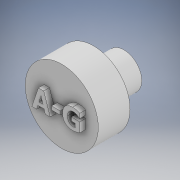
# Autodesk Inventor part: IPC A-G key
Saved by Autodesk Inventor 2022 (Build 260153000, 153)
## iProperties
Created: 2022-01-01
Part Number: IPC A-G key
Material: Generic
Document SubType Name: Modeling
Designer: solor
Density: 1 g/cm^3
Appearance: Default
Author: solor
Autodesk Inventor part; units mm, degrees
ref_plane "YZ Plane" through (0, 0, 0) normal (1, 0, 0) x (0, 1, 0)
ref_plane "XZ Plane" through (0, 0, 0) normal (0, 1, 0) x (-1, 0, 0)
ref_plane "XY Plane" through (0, 0, 0) normal (0, 0, 1) x (1, 0, 0)
sketch "Sketch1" plane through (0, 0, 0) normal (0, 0, 1) x (1, 0, 0)
  circle A0 centre (0, 0) radius 6.22 construction
  circle A1 centre (0, 0) radius 2.8
  line L0 (-0.675, 0.675) -> (-0.675, 2.025)
  line L1 (-0.675, 2.025) -> (0.675, 2.025)
  line L2 (0.675, 2.025) -> (0.675, 0.675)
  line L3 (0.675, 0.675) -> (2.025, 0.675)
  line L4 (2.025, 0.675) -> (2.025, -0.675)
  line L5 (2.025, -0.675) -> (0.675, -0.675)
  line L6 (0.675, -0.675) -> (0.675, -2.025)
  line L7 (0.675, -2.025) -> (-0.675, -2.025)
  line L8 (-0.675, -2.025) -> (-0.675, -0.675)
  line L9 (-0.675, -0.675) -> (-2.025, -0.675)
  line L10 (-2.025, -0.675) -> (-2.025, 0.675)
  line L11 (-2.025, 0.675) -> (-0.675, 0.675)
  circle A2 centre (0, 0) radius 5.75
  point P0 (-6.07, -6.1)
  dimension "d0" = 12.44
  dimension "d1" = 0.47
  constraints: 24 end point, 3 centre point, 1 coincident
  measures "d0" diameter of A0
  measures "d1" radial gap between concentric circles of A0 A2
extrude "Extrusion1" add sketch "Sketch1" along normal blind 5 contours A1 | L0 L1 L2 L3 L4 L5 L6 L7 L8 L9 L10 L11 | A2
extrude "Extrusion2" add sketch "Sketch1" against normal blind 4.8 contours A1
sketch "Sketch2" plane through (0, 0, 5) normal (0, 0, 1) x (1, 0, 0)
  point P0 (0, 0)
sketch "Sketch3" plane through (0, 0, 5) normal (0, 0, 1) x (1, 0, 0)
  line L0 (-3.7906, 1.642) -> (3.8677, 1.642) construction
  line L1 (3.8677, 1.642) -> (3.8677, -1.5876) construction
  line L2 (3.8677, -1.5876) -> (-3.7906, -1.5876) construction
  line L3 (-3.7906, -1.5876) -> (-3.7906, 1.642) construction
  line L4 (-3.803, -1.4674) -> (-2.7723, 1.5826)
  line L5 (-2.7723, 1.5826) -> (-1.9369, 1.5826)
  line L6 (-1.9369, 1.5826) -> (-0.9062, -1.4674)
  line L7 (-0.9062, -1.4674) -> (-1.6947, -1.4674)
  line L8 (-1.6947, -1.4674) -> (-1.885, -0.8445)
  line L9 (-1.885, -0.8445) -> (-2.844, -0.8445)
  line L10 (-2.844, -0.8445) -> (-3.0368, -1.4674)
  line L11 (-3.0368, -1.4674) -> (-3.803, -1.4674)
  line L12 (-2.0531, -0.2909) -> (-2.3645, 0.7176)
  line L13 (-2.3645, 0.7176) -> (-2.6784, -0.2909)
  line L14 (-2.6784, -0.2909) -> (-2.0531, -0.2909)
  line L15 (0.6633, -0.4046) -> (-0.6937, -0.4046)
  line L16 (-0.6937, -0.4046) -> (-0.6937, 0.1639)
  line L17 (-0.6937, 0.1639) -> (0.6633, 0.1639)
  line L18 (0.6633, 0.1639) -> (0.6633, -0.4046)
  spline S0 degree 2 poles (3.7528, -1.2944) (3.5526, -1.3759) (2.9125, -1.5316) (2.601, -1.5316) knots 0 0 0 1 2 2 2
  spline S1 degree 2 poles (2.601, -1.5316) (1.8818, -1.5316) (1.0291, -0.7012) (1.0291, 0.0601) knots 0 0 0 1 2 2 2
  spline S2 degree 2 poles (1.0291, 0.0601) (1.0291, 0.7769) (1.8818, 1.642) (2.6233, 1.642) knots 0 0 0 1 2 2 2
  spline S3 degree 2 poles (2.6233, 1.642) (3.0064, 1.642) (3.4859, 1.4961) (3.7405, 1.3725) knots 0 0 0 1 2 2 2
  line L19 (3.7405, 1.3725) -> (3.7405, 0.6558)
  line L20 (3.7405, 0.6558) -> (3.6712, 0.6558)
  spline S4 degree 2 poles (3.6712, 0.6558) (3.6169, 0.6978) (3.4093, 0.8584) (3.3104, 0.9128) knots 0 0 0 1 2 2 2
  spline S5 degree 2 poles (3.3104, 0.9128) (3.1967, 0.9796) (2.8952, 1.0735) (2.7271, 1.0735) knots 0 0 0 1 2 2 2
  spline S6 degree 2 poles (2.7271, 1.0735) (2.5318, 1.0735) (2.208, 0.9499) (2.082, 0.8238) knots 0 0 0 1 2 2 2
  spline S7 degree 2 poles (2.082, 0.8238) (1.9609, 0.7003) (1.82, 0.3221) (1.82, 0.0725) knots 0 0 0 1 2 2 2
  spline S8 degree 2 poles (1.82, 0.0725) (1.82, -0.4614) (2.3563, -0.9706) (2.8185, -0.9706) knots 0 0 0 1 2 2 2
  spline S9 degree 2 poles (2.8185, -0.9706) (2.8606, -0.9706) (2.9693, -0.9656) (3.0113, -0.9632) knots 0 0 0 1 2 2 2
  line L21 (3.0113, -0.9632) -> (3.0113, -0.3625)
  line L22 (3.0113, -0.3625) -> (2.4206, -0.3625)
  line L23 (2.4206, -0.3625) -> (2.4206, 0.2084)
  line L24 (2.4206, 0.2084) -> (3.7528, 0.2084)
  line L25 (3.7528, 0.2084) -> (3.7528, -1.2944)
  point P0 (0.0385, -1.5876)
  point P1 (3.8677, 0.0272)
  point P2 (0, 0.1089)
  point P3 (0, 0.1089)
  constraints: 2 midpoint, 2 other
extrude "Extrusion7" add sketch "Sketch3" along normal blind 0.9
body "Solid1"
